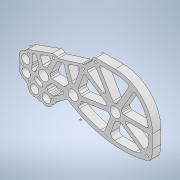
# Autodesk Inventor part: ギアマウント
Saved by Autodesk Inventor 2022.2 (Build 262287010, 287A)
## iProperties
Created: 2022-03-20
Part Number: ギアマウント
Material: Aluminum 2014-T6
Document SubType Name: Modeling
Designer: acps
Density: 2.78927 g/cm^3
Appearance: Satin
Author: acps
Autodesk Inventor part; units mm, degrees
ref_plane "YZ Plane" through (0, 0, 0) normal (1, 0, 0) x (0, 1, 0)
ref_plane "XZ Plane" through (0, 0, 0) normal (0, 1, 0) x (-1, 0, 0)
ref_plane "XY Plane" through (0, 0, 0) normal (0, 0, 1) x (1, 0, 0)
sketch "Sketch2" plane through (0, 0, 0) normal (0, 0, 1) x (1, 0, 0)
  line L0 (-44.2416, -60) -> (63.0185, -60) construction
  circle A0 centre (-30.6992, 12) radius 14 construction
  circle A1 centre (-44.5148, 14.4973) radius 14 construction
  circle A2 centre (-50.7402, 19.5218) radius 1.25
  circle A3 centre (-38.2895, 9.4728) radius 1.25
  circle A4 centre (-23.1088, 14.5272) radius 1.25
  circle A5 centre (-58.8465, 33.3162) radius 1.25
  circle A6 centre (-51.6122, 47.5873) radius 1.25
  circle A7 centre (-55.2294, 40.4518) radius 14 construction
  circle A8 centre (-54.7933, 26.419) radius 14 construction
  circle A9 centre (-33.8392, 34.0933) radius 22.3153 construction
  circle A10 centre (1.5644, 31.4) radius 30.9859 construction
  circle A11 centre (52, 38.9589) radius 41.9589 construction
  arc A12 (-55.772, 48.4584) -> (-53.0558, 51.5846) centre (-51.6122, 47.5873) ccw construction
  arc A13 (-62.5868, 35.3343) -> (-62.4543, 31.0698) centre (-58.8465, 33.3162) ccw
  circle A14 centre (-55.2294, 40.4518) radius 5.025
  arc A15 (-56.8528, 48.3109) -> (-62.528, 37.1155) centre (-55.2294, 40.4518) ccw
  circle A16 centre (-54.7933, 26.419) radius 5.025
  circle A17 centre (-54.7933, 26.419) radius 8.025
  circle A18 centre (-50.7402, 19.5218) radius 4.25 construction
  arc A19 (-36.8441, 5.4762) -> (-41.0426, 6.2351) centre (-38.2895, 9.4728) ccw construction
  arc A20 (-24.5543, 18.5238) -> (-21.87, 10.4617) centre (-23.1088, 14.5272) ccw construction
  circle A21 centre (-44.5148, 14.4973) radius 5.025
  circle A22 centre (-30.6992, 12) radius 5.025
  circle A23 centre (-44.5148, 14.4973) radius 8.025
  circle A24 centre (-30.6992, 12) radius 8.025
  arc A25 (-52.4687, 13.4308) -> (-57.0193, 18.7089) centre (-58.7877, 12.5834) ccw
  arc A26 (-41.0426, 6.2351) -> (-42.7724, 6.6637) centre (-42.3382, 4.7114) ccw
  arc A27 (-62.5868, 35.3343) -> (-62.528, 37.1155) centre (-64.347, 36.284) ccw
  arc A28 (-56.8528, 48.3109) -> (-55.451, 49.4112) centre (-57.2574, 50.2695) ccw
  arc A29 (-62.285, 29.2957) -> (-62.4543, 31.0698) centre (-64.1521, 30.0127) ccw
  arc A30 (-35.0737, 5.2721) -> (-36.8441, 5.4762) centre (-36.1639, 3.5954) ccw
  circle A31 centre (-21.8397, 58.0739) radius 1.5
  circle A32 centre (-21.8397, 58.0739) radius 4.5
  circle A33 centre (13.4218, 64.8462) radius 1.5
  circle A34 centre (13.4218, 64.8462) radius 4.5
  circle A35 centre (28.7706, 79.1935) radius 4.5
  circle A36 centre (28.7706, 79.1935) radius 1.5
  circle A37 centre (90.0569, 12.3112) radius 4.5
  circle A38 centre (90.0569, 12.3112) radius 1.5
  line L1 (-53.0558, 51.5846) -> (-23.3682, 62.3063)
  arc A39 (-18.3854, 60.958) -> (-16.2563, 60.33) centre (-16.8502, 62.2398) ccw
  line L2 (-16.2563, 60.33) -> (12.0856, 69.1432)
  circle A40 centre (-33.8392, 34.0933) radius 6.025
  circle A41 centre (-33.8392, 34.0933) radius 9.025
  arc A42 (-47.4788, 38.3562) -> (-31.6308, 19.9746) centre (-33.8392, 34.0933) ccw
  line L3 (-46.0723, 50.9171) -> (-28.4446, 57.2833)
  arc A43 (-25.942, 56.2243) -> (-28.4446, 57.2833) centre (-27.7652, 55.4023) ccw
  arc A44 (-24.9717, 52.9319) -> (-25.2463, 55.1336) centre (-26.7603, 53.8269) ccw
  line L4 (-24.9717, 52.9319) -> (-29.4813, 43.9197)
  arc A45 (-31.7359, 42.8698) -> (-29.4813, 43.9197) centre (-31.2699, 44.8147) ccw
  line L5 (-17.8154, 56.0602) -> (-25.8299, 40.0433)
  arc A46 (-25.8299, 40.0433) -> (-25.8187, 38.2313) centre (-24.0414, 39.1483) ccw
  line L6 (-33.8392, 34.0933) -> (-21.8397, 58.0739) construction
  line L7 (-47.4788, 38.3562) -> (-47.4212, 38.5991)
  line L8 (-47.2048, 40.5594) -> (-47.3924, 48.9915)
  arc A47 (-46.0723, 50.9171) -> (-47.3924, 48.9915) centre (-45.3929, 49.036) ccw
  line L9 (-54.7933, 26.419) -> (-33.8392, 34.0933) construction
  arc A48 (-48.1254, 34.4332) -> (-45.4382, 32.5076) centre (-46.126, 34.3856) ccw
  arc A49 (-43.7187, 27.8126) -> (-44.5266, 24.6069) centre (-43.0309, 25.9346) ccw
  arc A50 (-44.1499, 32.9795) -> (-42.8425, 34.7188) centre (-44.8377, 34.8575) ccw
  arc A51 (-40.3088, 27.8009) -> (-42.4303, 28.2844) centre (-41.7425, 26.4064) ccw
  line L10 (-45.4382, 32.5076) -> (-44.1499, 32.9795)
  line L11 (-43.7187, 27.8126) -> (-42.4303, 28.2844)
  line L12 (-33.8392, 34.0933) -> (-30.6992, 12) construction
  arc A52 (-34.8981, 23.7768) -> (-36.3269, 25.4179) centre (-36.8782, 23.4954) ccw
  arc A53 (-29.0328, 26.4546) -> (-29.9478, 24.4803) centre (-27.9677, 24.7618) ccw
  arc A54 (-37.1482, 20.1914) -> (-34.705, 22.4184) centre (-36.6851, 22.137) ccw
  arc A55 (-29.4846, 21.2209) -> (-28.1418, 19.6066) centre (-27.5045, 21.5023) ccw
  line L13 (-34.8981, 23.7768) -> (-34.705, 22.4184)
  line L14 (-29.9478, 24.4803) -> (-29.4846, 21.2209)
  arc A56 (-42.2975, 50.1539) -> (-44.858, 51.3557) centre (-44.1786, 49.4746) ccw
  arc A57 (-36.3931, 54.4127) -> (-37.5948, 51.8523) centre (-35.7137, 52.5317) ccw
  arc A58 (-40.1024, 40.5911) -> (-39.6093, 42.7105) centre (-41.4904, 42.0311) ccw
  arc A59 (-34.9066, 44.4088) -> (-33.1731, 43.0936) centre (-33.0255, 45.0882) ccw
  line L15 (-42.2975, 50.1539) -> (-39.6093, 42.7105)
  line L16 (-34.9066, 44.4088) -> (-37.5948, 51.8523)
  line L17 (-33.8392, 34.0933) -> (-40.6255, 52.8842) construction
  circle A60 centre (1.5644, 31.4) radius 6.025
  circle A61 centre (52, 38.9589) radius 6.025
  circle A62 centre (1.5644, 31.4) radius 10.025
  circle A63 centre (52, 38.9589) radius 9.025
  arc A64 (-16.6207, 57.075) -> (-17.8154, 56.0602) centre (-16.0268, 55.1652) ccw
  line L18 (-16.6207, 57.075) -> (6.788, 64.3542)
  arc A65 (9.2403, 63.1834) -> (6.788, 64.3542) centre (7.3818, 62.4444) ccw
  arc A66 (-26.3247, 18.7279) -> (-24.5543, 18.5238) centre (-25.2345, 20.4046) ccw
  arc A67 (-21.87, 10.4617) -> (-23.1648, 9.2372) centre (-21.287, 8.5486) ccw
  arc A68 (-22.4016, 18.7179) -> (-20.9398, 19.0391) centre (-22.0688, 20.69) ccw
  arc A69 (-18.1174, 14.9119) -> (-18.947, 13.6662) centre (-16.9884, 13.261) ccw
  line L19 (-20.9398, 19.0391) -> (-10.4193, 26.2336)
  arc A70 (-9.0516, 27.1689) -> (-8.2271, 29.249) centre (-10.1805, 28.8198) ccw construction
  arc A71 (-3.9917, 23.0555) -> (-6.2292, 23.0417) centre (-5.1002, 21.3908) ccw
  line L20 (-18.1174, 14.9119) -> (-6.2292, 23.0417)
  line L21 (-23.1088, 14.5272) -> (1.5644, 31.4) construction
  arc A72 (-25.3445, 37.1414) -> (-23.6137, 35.8226) centre (-23.462, 37.8168) ccw
  arc A73 (-23.993, 30.837) -> (-25.9033, 29.7952) centre (-24.1447, 28.8428) ccw
  arc A74 (-9.3651, 34.7387) -> (-7.4208, 35.8459) centre (-9.2134, 36.7329) ccw
  arc A75 (-7.99, 28.3644) -> (-9.7444, 29.7531) centre (-9.8961, 27.7588) ccw construction
  line L22 (-23.6137, 35.8226) -> (-9.3651, 34.7387)
  line L23 (-23.993, 30.837) -> (-11.3965, 29.8788)
  line L24 (-33.8392, 34.0933) -> (1.5644, 31.4) construction
  arc A76 (-10.4193, 26.2336) -> (-11.3965, 29.8788) centre (-11.5482, 27.8845) ccw
  line L25 (-11.3965, 29.8788) -> (-9.7444, 29.7531) construction
  line L26 (-10.4193, 26.2336) -> (-9.0516, 27.1689) construction
  line L27 (-7.319, 59.9675) -> (1.5644, 31.4) construction
  arc A77 (-9.1123, 57.3153) -> (-11.616, 58.6313) centre (-11.0221, 56.7215) ccw
  arc A78 (-3.0219, 61.3037) -> (-4.3379, 58.8) centre (-2.4281, 59.3939) ccw
  arc A79 (-4.7785, 39.1633) -> (-4.2408, 41.5776) centre (-6.0439, 40.7121) ccw
  arc A80 (0.6404, 42.7907) -> (2.3863, 41.3913) centre (2.5502, 43.3845) ccw construction
  line L28 (-9.1123, 57.3153) -> (-4.1341, 41.306)
  line L29 (-4.3379, 58.8) -> (-0.0658, 45.0619)
  arc A81 (-55.451, 49.4112) -> (-55.772, 48.4584) centre (-51.6122, 47.5873) ccw construction
  arc A82 (-55.772, 48.4584) -> (-56.8528, 48.3109) centre (-55.2294, 40.4518) ccw construction
  arc A83 (-62.528, 37.1155) -> (-62.0081, 36.1565) centre (-55.2294, 40.4518) ccw construction
  arc A84 (-62.0081, 36.1565) -> (-55.772, 48.4584) centre (-55.2294, 40.4518) ccw
  arc A85 (-62.0081, 36.1565) -> (-62.5868, 35.3343) centre (-58.8465, 33.3162) ccw construction
  arc A86 (-61.8257, 30.2852) -> (-62.0081, 36.1565) centre (-58.8465, 33.3162) ccw construction
  arc A87 (-62.4543, 31.0698) -> (-61.8257, 30.2852) centre (-58.8465, 33.3162) ccw
  arc A88 (-53.0558, 51.5846) -> (-55.451, 49.4112) centre (-51.6122, 47.5873) ccw
  arc A89 (-41.0426, 6.2351) -> (-36.8441, 5.4762) centre (-38.2895, 9.4728) ccw
  arc A90 (-22.4016, 18.7179) -> (-24.5543, 18.5238) centre (-23.1088, 14.5272) ccw
  arc A91 (-18.947, 13.6662) -> (-22.4016, 18.7179) centre (-23.1088, 14.5272) ccw construction
  arc A92 (-21.4252, 10.6249) -> (-18.947, 13.6662) centre (-23.1088, 14.5272) ccw
  arc A93 (-21.87, 10.4617) -> (-21.4252, 10.6249) centre (-23.1088, 14.5272) ccw
  arc A94 (10.2022, 36.488) -> (12.2219, 35.5252) centre (11.9255, 37.5031) ccw
  arc A95 (12.963, 30.5804) -> (11.3143, 29.0678) centre (13.2595, 28.6025) ccw
  arc A96 (41.6758, 39.9395) -> (43.306, 41.3807) centre (41.3794, 41.9174) ccw construction
  arc A97 (44.398, 34.0948) -> (42.4169, 34.9947) centre (42.7133, 33.0168) ccw
  line L30 (12.2219, 35.5252) -> (40.1519, 39.7111)
  line L31 (12.963, 30.5804) -> (42.4169, 34.9947)
  line L32 (1.5644, 31.4) -> (52, 38.9589) construction
  arc A98 (9.4982, 61.2607) -> (9.4005, 62.8266) centre (7.6132, 61.929) ccw
  arc A99 (15.2731, 60.7446) -> (14.2108, 59.59) centre (16.0959, 58.9217) ccw construction
  arc A100 (1.1349, 41.4158) -> (2.9342, 42.7457) centre (1.0492, 43.414) ccw construction
  arc A101 (7.6468, 41.0749) -> (8.2067, 38.9087) centre (9.5319, 40.4067) ccw
  line L33 (2.9342, 42.7457) -> (3.729, 44.9875) construction
  line L34 (14.2108, 59.59) -> (13.8416, 58.5486) construction
  line L35 (1.5644, 31.4) -> (13.4218, 64.8462) construction
  arc A102 (-0.0658, 45.0619) -> (3.729, 44.9875) centre (1.844, 45.6558) ccw
  line L36 (-0.0658, 45.0619) -> (0.6404, 42.7907) construction
  line L37 (3.729, 44.9875) -> (9.4982, 61.2607)
  line L38 (13.4218, 64.8462) -> (52, 38.9589) construction
  arc A103 (15.9236, 60.1567) -> (14.3823, 60.4499) centre (14.8092, 58.496) ccw construction
  arc A104 (17.8541, 65.6237) -> (18.7096, 64.3086) centre (19.824, 65.9693) ccw construction
  arc A105 (43.106, 40.4909) -> (42.2494, 42.4912) centre (41.135, 40.8304) ccw construction
  arc A106 (45.0355, 46.643) -> (47.2111, 46.6086) centre (46.1499, 48.3038) ccw construction
  line L39 (18.7096, 64.3086) -> (19.5182, 63.766) construction
  line L40 (42.2494, 42.4912) -> (40.9699, 43.3498) construction
  arc A107 (16.8411, 59.541) -> (13.8416, 58.5486) centre (15.7267, 57.8803) ccw
  line L41 (13.8416, 58.5486) -> (7.6468, 41.0749)
  line L42 (16.8411, 59.541) -> (15.9236, 60.1567) construction
  arc A108 (40.1519, 39.7111) -> (40.9699, 43.3498) centre (39.8555, 41.689) ccw
  line L43 (40.9699, 43.3498) -> (16.8411, 59.541)
  line L44 (40.1519, 39.7111) -> (41.6758, 39.9395) construction
  line L45 (28.7706, 79.1935) -> (52, 38.9589) construction
  line L46 (52, 38.9589) -> (90.0569, 12.3112) construction
  line L47 (52, 38.9589) -> (89.8711, 38.9589) construction
  arc A109 (-3.9917, 23.0555) -> (91.2724, 7.9784) centre (60.0574, 119.2475) ccw
  arc A110 (9.133, 21.1086) -> (76.1774, 9.8643) centre (60.0574, 119.2475) ccw
  arc A111 (8.6421, 24.3003) -> (9.133, 21.1086) centre (10.0541, 22.8838) ccw
  arc A112 (45.8797, 30.7071) -> (45.4475, 32.7528) centre (43.9954, 31.3775) ccw
  arc A113 (53.1598, 30.0087) -> (51.5326, 28.6958) centre (53.4169, 28.0253) ccw
  line L48 (45.8797, 30.7071) -> (40.253, 14.8928)
  line L49 (51.5326, 28.6958) -> (46.9075, 15.6968)
  arc A114 (34.3811, 11.7056) -> (40.253, 14.8928) centre (35.5423, 16.5689) ccw
  arc A115 (46.9075, 15.6968) -> (51.2185, 9.0367) centre (51.6182, 14.0207) ccw
  line L50 (41.7695, 10.2058) -> (52, 38.9589) construction
  arc A116 (13.6666, 69.3395) -> (15.1412, 69.8755) centre (13.7754, 71.3366) ccw
  arc A117 (18.5555, 66.2228) -> (17.9214, 64.7877) centre (19.9213, 64.7617) ccw construction
  line L51 (15.1412, 69.8755) -> (23.6368, 77.8169)
  arc A118 (23.6368, 77.8169) -> (24.2709, 79.252) centre (22.2711, 79.2779) ccw
  arc A119 (28.5258, 74.7001) -> (27.0512, 74.1642) centre (28.417, 72.7031) ccw construction
  line L52 (18.5555, 66.2228) -> (19.2669, 66.8878) construction
  line L53 (13.4218, 64.8462) -> (28.7706, 79.1935) construction
  arc A120 (19.2669, 66.8878) -> (19.5182, 63.766) centre (20.6327, 65.4267) ccw
  line L54 (19.2669, 66.8878) -> (26.3398, 73.4992)
  line L55 (19.5182, 63.766) -> (37.2955, 51.8368)
  arc A121 (28.9507, 73.8815) -> (27.6962, 74.8236) centre (27.2186, 72.8815) ccw construction
  arc A122 (44.6903, 44.2522) -> (44.8025, 46.4253) centre (43.0705, 45.4253) ccw construction
  line L56 (44.8025, 46.4253) -> (40.142, 54.4975) construction
  arc A123 (33.0922, 77.939) -> (33.2808, 76.3815) centre (35.0129, 77.3815) ccw construction
  arc A124 (49.1327, 48.9253) -> (51.0707, 47.9359) centre (50.8647, 49.9253) ccw
  line L57 (49.1327, 48.9253) -> (33.678, 75.6935)
  arc A125 (29.4376, 73.0381) -> (26.3398, 73.4992) centre (27.7055, 72.0381) ccw
  line L58 (26.3398, 73.4992) -> (27.0512, 74.1642) construction
  line L59 (29.4376, 73.0381) -> (28.9507, 73.8815) construction
  arc A126 (37.2955, 51.8368) -> (40.142, 54.4975) centre (38.41, 53.4975) ccw
  line L60 (40.142, 54.4975) -> (29.4376, 73.0381)
  line L61 (37.2955, 51.8368) -> (45.0355, 46.643) construction
  arc A127 (96.7346, 38.9589) -> (52, 83.6935) centre (52, 38.9589) ccw
  arc A128 (34.7706, 78.6935) -> (32.9244, 77.4627) centre (34.7706, 76.6935) ccw construction
  line L62 (28.7706, 83.6935) -> (52, 83.6935)
  line L63 (34.7706, 78.6935) -> (35.4101, 78.6935) construction
  arc A129 (35.4101, 78.6935) -> (33.678, 75.6935) centre (35.4101, 76.6935) ccw
  line L64 (35.4101, 78.6935) -> (52, 78.6935)
  line L65 (33.678, 75.6935) -> (33.2808, 76.3815) construction
  arc A130 (91.7346, 38.9589) -> (52, 78.6935) centre (52, 38.9589) ccw
  line L66 (91.7346, 38.9589) -> (91.7346, 27.8822)
  line L67 (96.7346, 38.9589) -> (96.7346, 22.9139)
  arc A131 (94.1926, 10.5375) -> (96.7346, 22.9139) centre (65.3346, 22.9139) ccw
  arc A132 (76.1774, 9.8643) -> (91.7346, 27.8822) centre (73.5221, 27.8822) ccw
  arc A133 (58.8107, 31.1381) -> (56.6361, 31.2157) centre (57.6635, 29.4998) ccw
  arc A134 (60.8619, 37.2507) -> (61.6786, 35.2338) centre (62.8257, 36.8721) ccw
  arc A135 (81.6082, 11.5632) -> (81.8674, 14.9936) centre (80.7202, 13.3553) ccw
  arc A136 (86.3221, 17.9782) -> (89.1898, 18.5969) centre (87.4693, 19.6165) ccw
  line L68 (58.8107, 31.1381) -> (81.8674, 14.9936)
  line L69 (61.6786, 35.2338) -> (86.3221, 17.9782)
  line L70 (52, 38.9589) -> (71.8673, 73.3701) construction
  arc A137 (52.4771, 47.9713) -> (54.3149, 48.9685) centre (52.5829, 49.9685) ccw
  arc A138 (59.5111, 45.9685) -> (59.5664, 43.8783) centre (61.2431, 44.9685) ccw
  arc A139 (68.1029, 72.8499) -> (67.1325, 75.6991) centre (66.3708, 73.8499) ccw
  arc A140 (76.2517, 70.4341) -> (73.299, 69.8499) centre (75.0311, 68.8499) ccw
  line L71 (68.1029, 72.8499) -> (54.3149, 48.9685)
  line L72 (59.5111, 45.9685) -> (73.299, 69.8499)
  line L73 (62.0648, 41.4589) -> (89.4653, 41.4589)
  line L74 (66.2722, 36.4589) -> (89.7346, 36.4589)
  arc A141 (66.2722, 36.4589) -> (65.125, 32.8206) centre (66.2722, 34.4589) ccw
  arc A142 (60.239, 42.6426) -> (62.0648, 41.4589) centre (62.0648, 43.4589) ccw
  arc A143 (89.4653, 41.4589) -> (91.451, 43.6974) centre (89.4653, 43.4589) ccw
  arc A144 (91.7346, 34.4589) -> (89.7346, 36.4589) centre (89.7346, 34.4589) ccw
  point P0 (0, 0)
  point P1 (0, 0)
  point P2 (-47.2064, 40.6303)
  point P3 (-47.537, 38.1651)
  dimension "d266" = 60
  dimension "d267" = 3
  dimension "d268" = 3
  dimension "d269" = 10.05
  dimension "d270" = 3
  dimension "d271" = 10.05
  dimension "d272" = 3
  dimension "d273" = 3
  dimension "d274" = 3
  dimension "d275" = 3
  dimension "d276" = 10.05
  dimension "d277" = 10.05
  dimension "d278" = 3
  dimension "d279" = 3
  dimension "d280" = 2
  dimension "d281" = 2
  dimension "d282" = 2
  dimension "d283" = 2
  dimension "d284" = 2
  dimension "d285" = 3
  dimension "d286" = 3
  dimension "d287" = 3
  dimension "d288" = 3
  dimension "d289" = 3
  dimension "d290" = 3
  dimension "d291" = 3
  dimension "d292" = 3
  dimension "d293" = 2
  dimension "d294" = 12.05
  dimension "d295" = 3
  dimension "d296" = 2
  dimension "d297" = 3
  dimension "d298" = 2
  dimension "d299" = 2
  dimension "d300" = 2
  dimension "d301" = 5
  dimension "d302" = 2
  dimension "d303" = 2
  dimension "d304" = 2
  dimension "d305" = 2
  dimension "d306" = 2
  dimension "d307" = 2.5
  dimension "d308" = 5
  dimension "d309" = 2
  dimension "d310" = 2
  dimension "d311" = 2
  dimension "d312" = 2
  dimension "d313" = 5
  dimension "d314" = 2.5
  dimension "d315" = 2
  dimension "d316" = 2
  dimension "d317" = 2
  dimension "d318" = 2
  dimension "d319" = 5
  dimension "d320" = 2.5
  dimension "d321" = 12.05
  dimension "d322" = 12.05
  dimension "d323" = 4
  dimension "d324" = 3
  dimension "d325" = 2
  dimension "d326" = 2
  dimension "d327" = 3
  dimension "d328" = 2
  dimension "d329" = 2
  constraints: 260 point on circle, 207 tangent, 150 end point, 137 centre point, 60 parallel, 8 point on line, 7 coincident, 7 horizontal, 3 concentric, 2 perpendicular, 2 vertical, 137 other
  measures "d266" distance from line of L0 point (0, 0)
  measures "d267" radial gap between concentric circles of A6 A12
  measures "d268" radial gap between concentric circles of A5 A13
  measures "d269" diameter of A14
  measures "d271" diameter of A16
  measures "d272" radial gap between concentric circles of A16 A17
  measures "d273" radial gap between concentric circles of A2 A18
  measures "d274" radial gap between concentric circles of A3 A19
  measures "d275" radial gap between concentric circles of A4 A20
  measures "d276" diameter of A21
  measures "d277" diameter of A22
  measures "d278" radial gap between concentric circles of A21 A23
  measures "d279" radial gap between concentric circles of A22 A24
  measures "d280" radius of A27
  measures "d281" radius of A28
  measures "d282" radius of A29
  measures "d283" radius of A26
  measures "d284" radius of A30
  measures "d285" diameter of A31
  measures "d286" radial gap between concentric circles of A31 A32
  measures "d287" diameter of A33
  measures "d288" diameter of A33
  measures "d289" diameter of A36
  measures "d290" radial gap between concentric circles of A36 A35
  measures "d291" diameter of A38
  measures "d292" radial gap between concentric circles of A38 A37
  measures "d293" radius of A39
  measures "d294" diameter of A40
  measures "d296" radius of A43
  measures "d297" distance between parallel lines of L1 L3
  measures "d298" radius of A44
  measures "d299" radius of A45
  measures "d300" radius of A46
  measures "d301" distance between parallel lines of L4 L5
  measures "d302" radius of A47
  measures "d303" radius of A48
  measures "d304" radius of A49
  measures "d305" radius of A50
  measures "d306" radius of A51
  measures "d307" distance between parallel lines of L10 L9
  measures "d308" distance between parallel lines of L11 L10
  measures "d309" radius of A52
  measures "d310" radius of A53
  measures "d311" radius of A54
  measures "d312" radius of A55
  measures "d313" distance between parallel lines of L14 L13
  measures "d314" distance between parallel lines of L13 L12
  measures "d315" radius of A56
  measures "d316" radius of A57
  measures "d317" radius of A58
  measures "d318" radius of A59
  measures "d319" distance between parallel lines of L16 L15
  measures "d320" distance between parallel lines of L15 L17
  measures "d321" diameter of A60
  measures "d322" diameter of A61
  measures "d325" radius of A64
  measures "d326" radius of A65
  measures "d327" distance between parallel lines of L18 L2
  measures "d328" radius of A66
  measures "d329" radius of A67
extrude "Extrusion1" add sketch "Sketch2" along normal blind 10 contours A2 A17 A23 A24 A3 | A2 A23 A17 | A23 A25 A17 A2 | A2 A17 A5 A84 A23 | A17 A42 A23 | A42 A24 A23 | A23 A3 A24 A30 A89 A26 | A17 A84 A42 | A42 A48 L10 A50 A41 A51 L11 A49 | A24 A4 A3 A23 | A23 A3 A24 | A54 L13 A52 A41 A53 L14 A55 A24 A42 | A29 A87 A17 | A84 A5 A17 | A17 A5 A87 A13 A27 A15 A28 A88 L1 A32 A43 L3 A47 L8 A84 | A66 A90 A68 L19 A76 L23 A73 A41 A72 L22 A74 A62 A71 L20 A69 A92 A93 A67 A24 A4 | A41 | A58 L15 A56 L3 A57 L16 A59 A41 | A45 L4 A44 A32 L5 A46 A41 | A32 | A39 L2 A34 A65 L18 A64 A32 | A62 | A62 A111 A110 A132 A37 A109 | A34 | A37 | A79 L28 A77 L18 A78 L29 A102 L37 A98 A34 A116 L51 A118 A35 L62 A127 L67 A131 A37 A132 L66 A130 L64 A129 L57 A124 A63 A97 L31 A95 A62 A94 L30 A108 L43 A107 L41 A101 | A132 A135 L68 A133 A63 A134 L69 A136 | A114 L48 A112 A63 A113 L49 A115 A110 | A35 | A63 | A144 L74 A141 L69 A134 A63 A142 L73 A143 A130 L66 | A137 L71 A139 A130 A140 L72 A138 A63 picked at (-49.1846, 20.8215) picked at (-37.9272, 13.1818) picked at (-54.9204, 33.1261)
body "Solid1"
